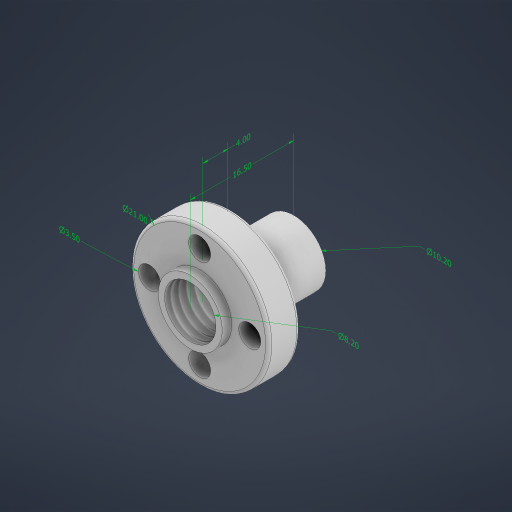
# Autodesk Inventor part: LeadNut
Saved by Autodesk Inventor 2024 (Build 280153000, 153)
## iProperties
Created: 2024-03-11
Part Number: LeadNut
Material: Generic
Document SubType Name: Modeling
Designer: LightStore
Density: 1 g/cm^3
Appearance: Default
Author: LightStore
Autodesk Inventor part; units mm, degrees
ref_plane "YZ Plane" through (0, 0, 0) normal (1, 0, 0) x (0, 1, 0)
ref_plane "XZ Plane" through (0, 0, 0) normal (0, 1, 0) x (-1, 0, 0)
ref_plane "XY Plane" through (0, 0, 0) normal (0, 0, 1) x (1, 0, 0)
sketch "Sketch1" plane through (0, 0, 0) normal (0, 0, 1) x (1, 0, 0)
  circle A0 centre (0, 0) radius 11
  circle A1 centre (0, 0) radius 8 construction
  line L0 (0, 0) -> (0, 8) construction
  circle A2 centre (0, 8) radius 1.75
  line L1 (0, 0) -> (-8, 0) construction
  circle A3 centre (-8, 0) radius 1.75
  line L2 (0, 0) -> (0, -8) construction
  circle A4 centre (0, -8) radius 1.75
  line L3 (0, 0) -> (8, 0) construction
  circle A5 centre (8, 0) radius 1.75
  dimension "d1" = 16
  dimension "d0" = 22
  dimension "d2" = 3.5
  dimension "d5" = 360
  constraints: 8 coincident, 8 end point, 5 centre point, 1 vertical alignment, 21 other
  measures "d0" diameter of A0
  measures "d2" diameter of A2
extrude "Extrusion1" add sketch "Sketch1" along normal blind 5
sketch "Sketch2" plane through (0, 0, 5) normal (0, 0, 1) x (1, 0, 0)
  circle A0 centre (0, 0) radius 5.1
  dimension "d10" = 10.2
  constraints: 1 centre point, 1 coincident
  measures "d10" diameter of A0
sketch "Sketch3" plane through (0, 0, 0) normal (0, 0, -1) x (-1, 0, 0)
  point P0 (0, 0)
extrude "Extrusion2" add sketch "Sketch2" along normal blind 1.5
sketch "Sketch4" plane through (0, 0, 0) normal (0, 0, -1) x (-1, 0, 0)
  circle A0 centre (0, 0) radius 5.1
  dimension "d13" = 10.2
  constraints: 1 centre point, 1 coincident
  measures "d13" diameter of A0
extrude "Extrusion3" add sketch "Sketch4" along normal blind 10
sketch "Sketch5" plane through (0, 0, 6.5) normal (0, 0, 1) x (1, 0, 0)
  circle A0 centre (0, 0) radius 4.1
  dimension "d16" = 8.2
  constraints: 1 centre point, 1 coincident
  measures "d16" diameter of A0
extrude "Extrusion4" cut sketch "Sketch5" against normal blind 19.5
thread "Thread1" size "M9x1.25" class "6H" standard "ANSI Metric M Profile" length 4000
fillet "Fillet1" radius 0.5 2 edges at (-11, 0, 5) (-11, 0, 0)
body "Solid1"
